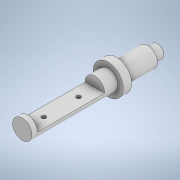
# Autodesk Inventor part: eixo da Valvula
Saved by Autodesk Inventor 2022 (Build 260153000, 153)
## iProperties
Created: 2022-06-22
Part Number: eixo da Valvula
Material: Genérico
Document SubType Name: Modeling
Designer: robofei
Density: 1 g/cm^3
Appearance: Padrão
Author: robofei
Autodesk Inventor part; units mm, degrees
ref_plane "YZ Plane" through (0, 0, 0) normal (1, 0, 0) x (0, 1, 0)
ref_plane "XY Plane" through (0, 0, 0) normal (0, 0, 1) x (1, 0, 0)
sketch "Esboço1" plane through (0, 0, 0) normal (0, 0, 1) x (1, 0, 0)
  circle A0 centre (0, 0) radius 18.75
  dimension "d2" = 37.5
  constraints: 1 centre point, 1 coincident
  measures "d2" diameter of A0
extrude "Extrusão1" add sketch "Esboço1" along normal blind 28.9
sketch "Esboço2" plane through (0, 0, 28.9) normal (0, 0, 1) x (1, 0, 0)
  circle A0 centre (0, 0) radius 28
  dimension "d3" = 56
  constraints: 1 centre point, 1 coincident
  measures "d3" diameter of A0
extrude "Extrusão2" add sketch "Esboço2" along normal blind 89.8
sketch "Esboço3" plane through (0, 0, 118.7) normal (0, 0, 1) x (1, 0, 0)
  circle A0 centre (0, 0) radius 43.6
  dimension "d6" = 87.2
  constraints: 1 centre point, 1 coincident
  measures "d6" diameter of A0
extrude "Extrusão3" add sketch "Esboço3" along normal blind 24
sketch "Esboço4" plane through (0, 0, 142.7) normal (0, 0, 1) x (1, 0, 0)
  circle A0 centre (0, 0) radius 28
  dimension "d9" = 56
  constraints: 1 centre point, 1 coincident
  measures "d9" diameter of A0
extrude "Extrusão4" add sketch "Esboço4" along normal blind 247.1
ref_plane "Plano de trabalho1" through (0, 28, 0) normal (0, 1, 0) x (-1, 0, 0)
sketch "Esboço5" plane through (0, 28, 0) normal (0, 1, 0) x (-1, 0, 0)
  line L0 (86.1192, 180.9) -> (-95.7284, 180.9)
  line L1 (-95.7284, 180.9) -> (-95.7284, 374.7)
  line L2 (-95.7284, 374.7) -> (86.1192, 374.7)
  line L3 (86.1192, 374.7) -> (86.1192, 180.9)
  line L4 (43.6, 142.7) -> (-43.6, 142.7) projected
  point P0 (0, 0)
  dimension "d13" = 193.8
  dimension "d14" = 38.2
  constraints: 8 end point, 2 parallel, 1 horizontal, 1 perpendicular
  measures "d13" distance of L0.end L1.end
  measures "d14" distance between parallel lines of L0 L4
extrude "Extrusão5" cut sketch "Esboço5" against normal blind 29
sketch "Esboço6" plane through (0, -1, 0) normal (0, 1, 0) x (1, 0, 0)
  circle A0 centre (0, -227.8) radius 6.25
  circle A1 centre (0, -327.8) radius 6.25
  line L0 (28, -180.9) -> (-28, -180.9) projected
  line L1 (-28, -374.7) -> (28, -374.7) projected
  point P0 (0, 0)
  point P1 (-27.9821, -180.9)
  point P2 (27.9821, -180.9)
  point P3 (27.9821, -374.7)
  point P4 (-27.9821, -374.7)
  dimension "d17" = 12.5
  dimension "d19" = 100
  dimension "d20" = 12.5
  dimension "d21" = 46.9
  constraints: 2 centre point
  measures "d17" diameter of A0
  measures "d19" distance of A1.centre A0.centre
  measures "d20" diameter of A1
  measures "d21" distance from line of L1 A1.centre
extrude "Extrusão6" cut sketch "Esboço6" against normal up to next
chamfer "Chanfro1" distance 1 angle 45 1 edges at (-18.75, 0, 0)
